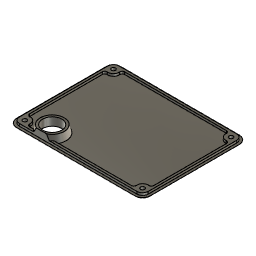
MainCaseTop (Autodesk Fusion 360 design; units mm, degrees)
Autodesk Fusion 360 part; units mm, degrees
sketch "Skizze1" plane through (0, 0, 0) normal (0, 0, 1) x (1, 0, 0)
  line L0 (50.5, -38) -> (-50.5, -38) construction
  line L1 (-50.5, -38) -> (-50.5, 38) construction
  line L2 (-50.5, 38) -> (50.5, 38) construction
  line L3 (50.5, 38) -> (50.5, -38) construction
  line L4 (50.5, -38) -> (-50.5, 38) construction
  line L5 (-50.5, -38) -> (50.5, 38) construction
  circle A0 centre (-50.5, 38) radius 4.8 construction
  circle A1 centre (-50.5, -38) radius 4.8 construction
  circle A2 centre (50.5, -38) radius 4.8 construction
  circle A3 centre (50.5, 38) radius 4.8 construction
  line L6 (-50.5, 45) -> (50.5, 45)
  line L7 (57.5, 38) -> (57.5, -38)
  line L8 (50.5, -45) -> (-50.5, -45)
  line L9 (-57.5, -38) -> (-57.5, 38)
  arc A4 (-50.5, 45) -> (-57.5, 38) centre (-50.5, 38) ccw
  arc A5 (-57.5, -38) -> (-50.5, -45) centre (-50.5, -38) ccw
  arc A6 (50.5, -45) -> (57.5, -38) centre (50.5, -38) ccw
  arc A7 (57.5, 38) -> (50.5, 45) centre (50.5, 38) ccw
  line L10 (-50.5, 42.8) -> (50.5, 42.8)
  line L11 (55.3, 38) -> (55.3, -37.9996)
  line L12 (50.5, -42.8) -> (-50.5, -42.8)
  line L13 (-55.3, -38) -> (-55.3, 38)
  line L14 (-53.3, 31.2472) -> (-53.3, -31.2472)
  line L15 (53.3, -31.2472) -> (53.3, 31.2472)
  line L16 (-43.7472, 40.8) -> (43.7472, 40.8)
  arc A8 (-51.0647, 33.2333) -> (-53.3, 31.2472) centre (-51.3, 31.2472) ccw
  arc A9 (-51.0647, 33.2333) -> (-45.7333, 38.5647) centre (-50.5, 38) ccw
  arc A10 (-43.7472, 40.8) -> (-45.7333, 38.5647) centre (-43.7472, 38.8) ccw
  arc A11 (50.5, -42.8) -> (55.3, -37.9996) centre (50.5, -38) ccw
  arc A12 (55.3, 38) -> (50.5, 42.8) centre (50.5, 38) ccw
  arc A13 (-55.3, -38) -> (-50.5, -42.8) centre (-50.5, -38) ccw
  arc A14 (-50.5, 42.8) -> (-55.3, 38) centre (-50.5, 38) ccw
  arc A15 (45.7333, 38.5647) -> (43.7472, 40.8) centre (43.7472, 38.8) ccw
  arc A16 (45.7333, 38.5647) -> (51.0647, 33.2333) centre (50.5, 38) ccw
  arc A17 (53.3, 31.2472) -> (51.0647, 33.2333) centre (51.3, 31.2472) ccw
  arc A18 (43.7472, -40.8) -> (45.7333, -38.5647) centre (43.7472, -38.8) ccw
  arc A19 (51.0647, -33.2333) -> (45.7333, -38.5647) centre (50.5, -38) ccw
  arc A20 (51.0647, -33.2333) -> (53.3, -31.2472) centre (51.3, -31.2472) ccw
  arc A21 (-45.7333, -38.5647) -> (-43.7472, -40.8) centre (-43.7472, -38.8) ccw
  arc A22 (-45.7333, -38.5647) -> (-51.0647, -33.2333) centre (-50.5, -38) ccw
  arc A23 (-53.3, -31.2472) -> (-51.0647, -33.2333) centre (-51.3, -31.2472) ccw
  circle A24 centre (-50.5, -38) radius 1.75
  circle A25 centre (-50.5, 38) radius 1.75
  circle A26 centre (50.5, 38) radius 1.75
  circle A27 centre (50.5, -38) radius 1.75
  circle A28 centre (-31.5, -33.5) radius 8.25
  arc A29 (-27.1904, -42.8) -> (-35.8096, -42.8) centre (-31.5, -33.5) ccw
  line L17 (-43.7472, -40.8) -> (-35.3435, -40.8)
  line L18 (-27.6565, -40.8) -> (43.7472, -40.8)
  dimension "d1" = 101
  dimension "d2" = 76
  dimension "d3" = 9.6
  dimension "d4" = 7
  dimension "d5" = 7
  dimension "d6" = 7
  dimension "d7" = 7
  dimension "d10" = 2
  dimension "d11" = 2
  dimension "d12" = 2
  dimension "d13" = 2
  dimension "d14" = 2
  dimension "d15" = 3.5
  dimension "d16" = 33.5
  dimension "d17" = 31.5
  dimension "d18" = 16.5
  dimension "d19" = 2
  constraint horizontal L0
  constraint perpendicular L0 L1
  constraint parallel L0 L2
  constraint parallel L1 L3
  constraint coincident L4 origin
  constraint coincident L5 origin
  constraint coincident L1.end L2.start
  constraint coincident L0.end L1.start
  constraint coincident L0.start L3.end
  constraint coincident L2.end L3.start
  constraint equal A0 A3
  constraint equal A0 A1
  constraint equal A1 A2
  constraint horizontal L6
  constraint vertical L7
  constraint horizontal L8
  constraint vertical L9
  constraint tangent L6 A4
  constraint tangent L9 A4
  constraint tangent L9 A5
  constraint tangent L8 A5
  constraint tangent L8 A6
  constraint tangent L7 A6
  constraint tangent L7 A7
  constraint tangent L6 A7
  constraint coincident A0 L10.start
  constraint coincident A3 L10.end
  constraint parallel L2 L10
  constraint coincident A3 L11.start
  constraint coincident A2 L11.end
  constraint perpendicular L10 L11
  constraint coincident A2 L12.start
  constraint coincident A1 L12.end
  constraint perpendicular L11 L12
  constraint coincident A1 L13.start
  constraint coincident A0 L13.end
  constraint perpendicular L12 L13
  constraint tangent A0 L13
  constraint tangent A0 L10
  constraint tangent A3 L11
  constraint tangent A2 L12
  constraint parallel L1 L14
  constraint horizontal L17
  constraint vertical L15
  constraint horizontal L16
  constraint tangent L14 A8
  constraint tangent A8 A9
  constraint tangent A9 A10
  constraint coincident L16.start A10.start
  constraint tangent L16 A10
  constraint equal A0 A9
  constraint tangent L12 A11
  constraint tangent L11 A12
  constraint tangent L12 A13
  constraint tangent L13 A14
  constraint equal A8 A10
  constraint tangent L16 A15
  constraint tangent A15 A16
  constraint tangent A16 A17
  constraint equal A3 A16
  constraint equal A10 A15
  constraint equal A15 A17
  constraint tangent L15 A17
  constraint tangent A18 L17
  constraint tangent A18 A19
  constraint tangent A19 A20
  constraint equal A17 A20
  constraint equal A2 A19
  constraint equal A18 A20
  constraint coincident L15.start A20.end
  constraint tangent L15 A20
  constraint tangent A21 L17
  constraint tangent A21 A22
  constraint tangent A22 A23
  constraint equal A1 A22
  constraint equal A18 A21
  constraint equal A21 A23
  constraint tangent L14 A23
  constraint concentric A1 A24
  constraint concentric A4 A25
  constraint concentric A16 A26
  constraint concentric A6 A27
  constraint equal A24 A25
  constraint equal A25 A26
  constraint equal A26 A27
  constraint coincident L12 A29.start
  constraint coincident L12 A29.end
  constraint coincident A28.centre A29.centre
  constraint coincident A28 L17.end
  constraint coincident A28 L18.start
  constraint collinear L17 L18
  measures "d1" distance of L1.end L2.end
  measures "d2" distance of L0.end L1.end
  measures "d3" diameter of A0
  measures "d4" radius of A4
  measures "d5" radius of A5
  measures "d6" radius of A6
  measures "d7" radius of A7
  measures "d10" distance of L13 L14
  measures "d11" distance of L10 L16
  measures "d12" radius of A8
  measures "d13" distance of L11 L15
  measures "d14" distance of L12 L17
  measures "d15" diameter of A24
  measures "d16" vertical distance of origin A28.centre
  measures "d17" horizontal distance of origin A28.centre
  measures "d18" diameter of A28
  measures "d19" distance of A28 A29
extrude "Extrusion1" add sketch "Skizze1" against normal blind 1 contours L6 L7 L8 L9 A4 A5 A6 A7 | L10 L11 L12 L13 L14 L15 L16 A8 A9 A10 A11 A12 A13 A14 A15 A16 A17 A18 A19 A20 A21 A22 A23 A29 L17 L18 | L12 A28 A29 L17 L18 | L14 L15 L16 A8 A9 A10 A15 A16 A17 A18 A19 A20 A21 A22 A23 A29 L17 L18 | A28 A29 L17 L18
extrude "Extrusion2" add sketch "Skizze1" along normal blind 2 contours L10 L11 L12 L13 L14 L15 L16 A8 A9 A10 A11 A12 A13 A14 A15 A16 A17 A18 A19 A20 A21 A22 A23 A29 L17 L18
extrude "Extrusion3" add sketch "Skizze1" along normal blind 6 contours L12 A28 A29 L17 L18 | A28 A29 L17 L18
chamfer "Fase2" distance 1 angle 45 8 edges at (0, -45, -1) (-55.4497, -42.9497, -1) (-57.5, 0, -1) (-55.4497, 42.9497, -1) (0, 45, -1) (55.4497, 42.9497, -1) (57.5, 0, -1) (55.4497, -42.9497, -1)
draft "Verjüngung2" angle 15.95 neutral plane through (0, 0, 6) pull (0, 0, 1) 1 faces at (-30.746, -23.2778, 2)
